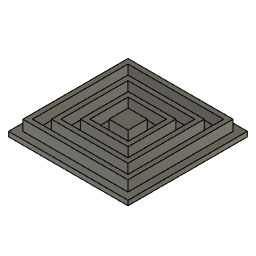
square_triple_2mm_ v2 (Autodesk Fusion 360 design; units mm, degrees)
Autodesk Fusion 360 part; units mm, degrees
sketch "Sketch1" plane through (0, 0, 0) normal (0, 0, 1) x (1, 0, 0)
  line L0 (0, 0) -> (25, 0)
  line L1 (25, 0) -> (25, 25)
  line L2 (25, 25) -> (0, 25)
  line L3 (0, 25) -> (0, 0)
  dimension "d1" = 25
  dimension "d2" = 25
  constraint horizontal L0
  constraint vertical L1
  constraint horizontal L2
  constraint vertical L3
  constraint coincident L0.start L3.end
  measures "d1" distance of L0.start L0.end
  measures "d2" distance of L0.start L2.end
extrude "Extrude1" add sketch "Sketch1" along normal blind 1
sketch "Sketch12" plane through (0, 0, 1) normal (0, 0, 1) x (-1, 0, 0)
  line L0 (0, -25) -> (0, 0)
  line L1 (0, 0) -> (-25, 0)
  line L2 (-25, 0) -> (-25, -25)
  line L3 (-25, -25) -> (0, -25)
  line L4 (-1.503, -1.4918) -> (-23.503, -1.4918)
  line L5 (-23.503, -1.4918) -> (-23.503, -23.4918)
  line L6 (-23.503, -23.4918) -> (-1.503, -23.4918)
  line L7 (-1.503, -23.4918) -> (-1.503, -1.4918)
  dimension "d54" = 22
  dimension "d55" = 22
  constraint horizontal L4
  constraint vertical L5
  constraint horizontal L6
  constraint vertical L7
  measures "d54" distance of L4.start L4.end
  measures "d55" distance of L4.start L6.end
extrude "Extrude15" add sketch "Sketch12" along normal blind 2.2 contours L4 L5 L6 L7
shell "Shell5" thickness 1 removed faces 1 at (8.8363, 16.1585, 3.2)
sketch "Sketch7" plane through (0, 0, 1) normal (0, 0, 1) x (-1, 0, 0)
  line L0 (0, -25) -> (0, 0)
  line L1 (0, 0) -> (-25, 0)
  line L2 (-25, 0) -> (-25, -25)
  line L3 (-25, -25) -> (0, -25)
  line L4 (-4.4883, -20.4835) -> (-20.4883, -20.4835)
  line L5 (-20.4883, -20.4835) -> (-20.4883, -4.4835)
  line L6 (-20.4883, -4.4835) -> (-4.4883, -4.4835)
  line L7 (-4.4883, -4.4835) -> (-4.4883, -20.4835)
  line L8 (-1.503, -23.4918) -> (-23.503, -23.4918)
  line L9 (-23.503, -23.4918) -> (-23.503, -1.4918)
  line L10 (-23.503, -1.4918) -> (-1.503, -1.4918)
  line L11 (-1.503, -1.4918) -> (-1.503, -23.4918)
  dimension "d22" = 16
  dimension "d23" = 16
  constraint horizontal L4
  constraint vertical L5
  constraint horizontal L6
  constraint vertical L7
  measures "d22" distance of L4.start L4.end
  measures "d23" distance of L4.start L6.end
extrude "Extrude5" add sketch "Sketch7" along normal blind 2.2 contours L4 L5 L6 L7
shell "Shell2" thickness 1 removed faces 1 at (9.8217, 15.1501, 3.2)
sketch "Sketch8" plane through (0, 0, 1) normal (0, 0, 1) x (-1, 0, 0)
  line L0 (-5.4883, -5.4835) -> (-19.4883, -5.4835)
  line L1 (-19.4883, -5.4835) -> (-19.4883, -19.4835)
  line L2 (-19.4883, -19.4835) -> (-5.4883, -19.4835)
  line L3 (-5.4883, -19.4835) -> (-5.4883, -5.4835)
  line L4 (-7.5145, -17.518) -> (-17.5145, -17.518)
  line L5 (-17.5145, -17.518) -> (-17.5145, -7.518)
  line L6 (-17.5145, -7.518) -> (-7.5145, -7.518)
  line L7 (-7.5145, -7.518) -> (-7.5145, -17.518)
  dimension "d27" = 10
  dimension "d28" = 10
  constraint horizontal L4
  constraint vertical L5
  constraint horizontal L6
  constraint vertical L7
  measures "d27" distance of L4.start L4.end
  measures "d28" distance of L4.start L6.end
extrude "Extrude6" add sketch "Sketch8" along normal blind 2.2 contours L4 L5 L6 L7
shell "Shell3" thickness 1 removed faces 1 at (10.8478, 14.1847, 3.2)
sketch "Sketch9" plane through (0, 0, 1) normal (0, 0, 1) x (-1, 0, 0)
  line L0 (-8.5145, -8.518) -> (-16.5145, -8.518)
  line L1 (-16.5145, -8.518) -> (-16.5145, -16.518)
  line L2 (-16.5145, -16.518) -> (-8.5145, -16.518)
  line L3 (-8.5145, -16.518) -> (-8.5145, -8.518)
  line L4 (-10.4987, -14.5206) -> (-14.4987, -14.5206)
  line L5 (-14.4987, -14.5206) -> (-14.4987, -10.5206)
  line L6 (-14.4987, -10.5206) -> (-10.4987, -10.5206)
  line L7 (-10.4987, -10.5206) -> (-10.4987, -14.5206)
  dimension "d32" = 4
  dimension "d33" = 4
  constraint horizontal L4
  constraint vertical L5
  constraint horizontal L6
  constraint vertical L7
  measures "d32" distance of L4.start L4.end
  measures "d33" distance of L4.start L6.end
extrude "Extrude7" add sketch "Sketch9" along normal blind 2.2 contours L4 L5 L6 L7
